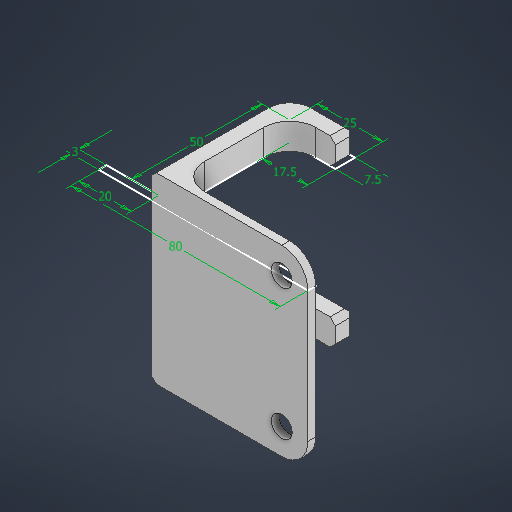
# Autodesk Inventor part: Hook
Saved by Autodesk Inventor 2026.2 (Build 302298000, 298)
## iProperties
Created: 2025-12-30
Part Number: Hook
Material: Generic
Document SubType Name: Modeling
Designer: Cobble
Density: 1 g/cm^3
Appearance: Default
Author: Cobble
Autodesk Inventor part; units mm, degrees
ref_plane "YZ Plane" through (0, 0, 0) normal (1, 0, 0) x (0, 1, 0)
ref_plane "XZ Plane" through (0, 0, 0) normal (0, 1, 0) x (-1, 0, 0)
ref_plane "XY Plane" through (0, 0, 0) normal (0, 0, 1) x (1, 0, 0)
sketch "Sketch1" plane through (0, 0, 0) normal (0, 0, 1) x (1, 0, 0)
  line L0 (0, 0) -> (0, 50)
  line L1 (0, 50) -> (25, 50)
  line L2 (25, 50) -> (25, 42.5)
  line L3 (25, 42.5) -> (7.5, 42.5)
  line L4 (7.5, 42.5) -> (7.5, 0)
  line L5 (7.5, 0) -> (0, 0)
  line L6 (0, 0) -> (-20, 0)
  line L7 (-20, 0) -> (-20, -3)
  line L8 (-20, -3) -> (60, -3)
  line L9 (60, -3) -> (60, 0)
  line L10 (60, 0) -> (7.5, 0)
  line L11 (0, 0) -> (0, -3)
  dimension "d0" = 50
  dimension "d1" = 25
  dimension "d2" = 7.5
  dimension "d3" = 17.5
  dimension "d4" = 20
  dimension "d5" = 3
  dimension "d6" = 80
  constraints: 24 end point, 10 perpendicular, 3 point on line, 1 vertical
  measures "d0" distance of L0.start L0.end
  measures "d1" distance of L0.end L1.end
  measures "d2" distance of L1.end L2.end
  measures "d3" distance of L2.end L3.end
  measures "d4" distance of L0.start L6.end
  measures "d5" distance of L6.end L7.end
  measures "d6" distance of L7.end L8.end
extrude "Extrusion1" add sketch "Sketch1" along normal blind 10 contours L5 L10 L9 L8 L11
extrude "Extrusion2" add sketch "Sketch1" along normal blind 10 contours L0 L1 L2 L3 L4 L5
extrude "Extrusion3" add sketch "Sketch1" against normal blind 60 contours L5 L10 L9 L8 L11
extrude "Extrusion4" add sketch "Sketch1" against normal blind 60 contours L0 L1 L2 L3 L4 L5
extrude "Extrusion5" cut sketch "Sketch1" against normal blind 50 contours L0 L1 L2 L3 L4 L5
fillet "Fillet1" radius 10 5 edges at (60, -1.5, 10) (60, -1.5, -60) (7.5, 0, 5) (7.5, 42.5, 5) (7.5, 42.5, -55)
fillet "Fillet2" radius 10 2 edges at (0, 50, -55) (0, 50, 5)
chamfer "Chamfer1" distance 2 angle 45 12 edges at (0, 18.5, -60) (2.9289, 47.0711, -60) (17.5, 50, -60) (0, 18.5, 10) (2.9289, 47.0711, 10) (17.5, 50, 10) (0, 20, -50) (2.9289, 47.0711, -50) (17.5, 50, -50) (0, 20, 0) (2.9289, 47.0711, 0) (17.5, 50, 0)
chamfer "Chamfer2" distance 2 angle 45 6 edges at (25, 45.25, -60) (25, 50, -55) (25, 45.25, -50) (25, 45.25, 0) (25, 45.25, 10) (25, 50, 5)
sketch "Sketch2" plane through (17.5, 0, 10) normal (0, 1, 0) x (1, 0, 0)
  arc A0 (32.5, 0) -> (42.5, 10) centre (32.5, 10) ccw projected
  arc A1 (42.5, 60) -> (32.5, 70) centre (32.5, 60) ccw projected
  circle A2 centre (32.5, 10) radius 4
  circle A3 centre (32.5, 60) radius 4
  point P0 (-17.5, 10)
  dimension "d25" = 8
  dimension "d26" = 8
  constraints: 2 centre point, 2 coincident
  measures "d25" diameter of A2
  measures "d26" diameter of A3
extrude "Extrusion6" cut sketch "Sketch2" against normal blind 60
body "Solid1"
